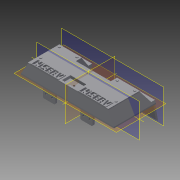
# Autodesk Inventor part: ChassisHintenUnten
Saved by Autodesk Inventor 2015 (Build 190159000, 159)
## iProperties
Created: 2018-11-28
Part Number: ChassisHintenUnten
Material: Generisch
Document SubType Name: Modeling
Designer: Boris
Density: 1 g/cm^3
Appearance: Vorgabe
Author: Boris
Autodesk Inventor part; units mm, degrees
sketch "Skizze1" plane through (0, 0, 0) normal (0, 0, 1) x (1, 0, 0)
  line L0 (-76, 34.5) -> (76, 34.5)
  line L1 (76, 34.5) -> (76, -34.5)
  line L2 (76, -34.5) -> (-76, -34.5)
  line L3 (-76, -34.5) -> (-76, 34.5)
  line L4 (0, -48.3) -> (0, 48.3) projected
  line L5 (-106.4, 0) -> (106.4, 0) projected
  point P0 (0, 0)
  dimension "d0" = 69
  dimension "d1" = 152
  constraints: 8 end point, 2 parallel, 1 horizontal, 1 perpendicular, 2 other
  measures "d0" distance of L0.end L1.end
  measures "d1" distance of L1.end L2.end
extrude "Extrusion1" add sketch "Skizze1" along normal blind 20
sketch "Skizze2" plane through (0, 0, 20) normal (0, 0, 1) x (1, 0, 0)
  line L0 (-76, 34.5) -> (-76, -34.5) projected
  line L1 (-76, -34.5) -> (76, -34.5) projected
  line L2 (76, -34.5) -> (76, 34.5) projected
  line L3 (-74.5, 34.5) -> (-74.5, -33)
  line L4 (-74.5, -33) -> (74.5, -33)
  line L5 (74.5, -33) -> (74.5, 34.5)
  line L6 (-76, 34.5) -> (-74.5, 34.5)
  line L7 (76, 34.5) -> (-76, 34.5) projected
  line L8 (74.5, 34.5) -> (76, 34.5)
  point P0 (0, 0)
  dimension "d4" = 1.5
  constraints: 10 end point, 1 collinear, 1 horizontal, 2 other
  measures "d4" distance between parallel lines of L0 L3
extrude "Extrusion2" cut sketch "Skizze2" against normal blind 20 contours L6 L3 L4 L5 L7 L2 L1 L0
sketch "Skizze4" plane through (0, 0, 20) normal (0, 0, 1) x (1, 0, 0)
  line L0 (-74.5, 34.5) -> (-74.5, -33) projected
  line L1 (-74.5, -33) -> (74.5, -33) projected
  line L2 (74.5, -33) -> (74.5, 34.5) projected
  line L3 (74.5, 34.5) -> (-74.5, 34.5) projected
  line L4 (-74.5, 34.5) -> (74.5, 34.5)
  line L5 (74.5, 34.5) -> (74.5, 28.5)
  line L6 (74.5, 28.5) -> (-74.5, 28.5)
  line L7 (-74.5, 28.5) -> (-74.5, 34.5)
  point P0 (0, 0)
  dimension "d10" = 6
  constraints: 8 end point, 2 parallel, 1 horizontal, 1 perpendicular, 1 point on line
  measures "d10" distance of L4.end L5.end
extrude "Extrusion4" cut sketch "Skizze4" against normal blind 15 contours L3 L2 L6 L0
chamfer "Fase1" distance 10 distance2 15 1 edges at (0, 28.5, 20) measured on face at (0, 28, 20)
chamfer "Fase2" distance 1 distance2 18 1 edges at (0, -33, 20) measured on face at (0, -32.5, 20)
sketch "Skizze5" plane through (-76, -34.5, 0) normal (-1, 0, 0) x (0, 0, 1)
  line L0 (0, 88.3544) -> (0, -14.7257) projected
  line L1 (0, 69) -> (-26.5167, 73.8189)
  line L2 (0, 69) -> (26.951, 69) construction
  line L3 (-26.5167, 73.8189) -> (-23.2032, 70.2167)
  line L4 (-26.5167, 73.8189) -> (-22.013, 73.8189) construction
  line L5 (0, 69) -> (0, 66)
  line L6 (0, 0) -> (0, 69) projected
  line L7 (0, 66) -> (-23.2032, 70.2167)
  point P0 (0, 34.5)
  dimension "d19" = 169.7
  dimension "d21" = 26.951
  dimension "d22" = 47.39
  dimension "d23" = 3
  constraints: 12 end point, 2 horizontal, 1 equal length, 1 parallel, 1 point on line
  measures "d19" angle of L2 L1
  measures "d21" distance of L1.start L1.end
  measures "d22" angle of L3 L4
  measures "d23" distance of L1.start L5.end
extrude "Extrusion5" add sketch "Skizze5" against normal up to surface (152 mm away)
fillet "Rundung1" radius 2 1 edges at (0, 31.5, 0)
sketch "Skizze6" plane through (0, 0, 20) normal (0, 0, 1) x (1, 0, 0)
  line L0 (-28, 46.7837) -> (28, 46.7837)
  line L1 (28, 46.7837) -> (28, 8.5)
  line L2 (28, 8.5) -> (-28, 8.5)
  line L3 (-28, 8.5) -> (-28, 46.7837)
  line L4 (0, 63.0404) -> (0, -50.7567) projected
  line L5 (-74.5, 18.5) -> (74.5, 18.5) projected
  point P0 (0, 0)
  dimension "d27" = 56
  dimension "d28" = 10
  constraints: 8 end point, 2 parallel, 1 horizontal, 1 perpendicular, 1 other
  measures "d27" distance of L1.end L2.end
  measures "d28" distance between parallel lines of L2 L5
extrude "Extrusion6" cut sketch "Skizze6" against normal blind 10
chamfer "Fase3" distance 10 distance2 18 1 edges at (74.5, -6.75, 20) measured on face at (74, -6.75, 20)
chamfer "Fase4" distance 10 distance2 18 1 edges at (-74.5, -6.75, 20) measured on face at (-74, -6.75, 20)
sketch "Skizze7" plane through (0, 0, 0) normal (0, 0, -1) x (-1, 0, 0)
  line L0 (-74.5, 29.8307) -> (74.5, 29.8307) projected
  line L1 (69, 22.8307) -> (-69, 22.8307)
  line L2 (-69, 22.8307) -> (-69, -27.5)
  line L3 (-69, -27.5) -> (69, -27.5)
  line L4 (69, -27.5) -> (69, 22.8307)
  line L5 (-74.5, 29.8307) -> (-74.5, -33) projected
  line L6 (-74.5, -33) -> (74.5, -33) projected
  line L7 (74.5, -33) -> (74.5, 29.8307) projected
  point P0 (0, 0)
  dimension "d37" = 7
  constraints: 8 end point
  measures "d37" distance between parallel lines of L0 L1
extrude "Extrusion7" cut sketch "Skizze7" against normal blind 10 contours L4 L3 L2 L1
sketch "Skizze8" plane through (0, 0, 10) normal (0, 0, -1) x (-1, 0, 0)
  line L0 (60.5, -27.5) -> (-60.5, -27.5)
  line L1 (-60.5, -32) -> (-60.5, 14.5)
  line L2 (-60.5, 14.5) -> (-32, 14.5)
  line L3 (-32, 14.5) -> (-32, 4.5)
  line L4 (-32, 4.5) -> (32, 4.5)
  line L5 (32, 4.5) -> (32, 14.5)
  line L6 (32, 14.5) -> (60.5, 14.5)
  line L7 (60.5, 14.5) -> (60.5, -32)
  point P0 (0, 0)
  point P1 (-28, 18.5)
  point P2 (28, 8.5)
  point P3 (-64.5, 28.5)
  point P4 (64.5, 28.5)
  constraints: 16 end point, 2 point on line
extrude "Extrusion8" cut sketch "Skizze8" against normal blind 4
sketch "Skizze9" plane through (0, 0, 10) normal (0, 0, 1) x (1, 0, 0)
  line L0 (-28, 8.5) -> (-28, 25.1667) projected
  line L1 (-28, 18.5) -> (28, 18.5)
  line L2 (28, 18.5) -> (28, 68.5)
  line L3 (28, 68.5) -> (-28, 68.5)
  line L4 (-28, 68.5) -> (-28, 18.5)
  line L5 (28, 8.5) -> (-28, 8.5) projected
  point P0 (0, 0)
  point P1 (-28, 28.5)
  dimension "d43" = 56
  dimension "d44" = 50
  dimension "d47" = 10
  constraints: 8 end point, 2 parallel, 1 horizontal, 1 perpendicular, 1 point on line
  measures "d43" distance of L3.end L2.end
  measures "d44" distance of L2.end L1.end
  measures "d47" distance between parallel lines of L5 L1
extrude "Extrusion9" cut sketch "Skizze9" against normal blind 60
sketch "Skizze10" plane through (0, 0, 0) normal (0, 0, -1) x (-1, 0, 0)
  line L0 (0, -48.3) -> (0, 48.3) projected
  line L1 (-40, -29.55) -> (-20, -29.55)
  line L2 (-20, -29.55) -> (-20, -32.45)
  line L3 (-20, -32.45) -> (-40, -32.45)
  line L4 (-40, -32.45) -> (-40, -29.55)
  point P0 (0, 0)
  dimension "d48" = 20
  dimension "d49" = 2.9
  dimension "d50" = 20
  constraints: 8 end point, 2 parallel, 1 horizontal, 1 perpendicular
  measures "d48" distance of L2.end L3.end
  measures "d49" distance of L1.end L2.end
  measures "d50" distance between parallel lines of L0 L2
extrude "Extrusion10" add sketch "Skizze10" along normal blind 15
fillet "Rundung2" radius 2 2 edges at (40, -31, -15) (20, -31, -15)
sketch "Skizze11" plane through (20, -29.55, 0) normal (0, 1, 0) x (1, 0, 0)
  circle A0 centre (15, 7.5) radius 1.5
  line L0 (20, 0) -> (0, 0) projected
  line L1 (20, 0) -> (20, 13) projected
  line L2 (2, 15) -> (18, 15) projected
  line L3 (10, 15) -> (10, 0)
  circle A1 centre (5, 7.5) radius 1.5
  point P0 (-20, 0)
  dimension "d55" = 3
  dimension "d56" = 7.5
  dimension "d57" = 5
  constraints: 2 centre point, 2 end point, 2 midpoint, 1 symmetric about line, 1 other
  measures "d55" diameter of A0
  measures "d56" distance from line of L0 A0.centre
  measures "d57" distance from line of A0.centre L1
extrude "Extrusion11" cut sketch "Skizze11" against normal blind 15
thread "Gewinde1" size "M3x0.5" class "6H" standard "ANSI Metric M Profile" full length
thread "Gewinde2" size "M3x0.5" class "6H" standard "ANSI Metric M Profile" full length
mirror "Spiegeln1" about plane through (0, 0, 0) normal (1, 0, 0) of "Extrusion10", "Rundung2", "Extrusion11"
sketch "Skizze12" plane through (0, 0, 20) normal (0, 0, 1) x (1, 0, 0)
  line L0 (-64.5, -32) -> (-64.5, 18.5) projected
  line L1 (64.5, -32) -> (-64.5, -32) projected
  line L2 (64.5, 18.5) -> (64.5, -32) projected
  line L3 (28, 18.5) -> (28, 8.5) projected
  line L4 (28, 8.5) -> (-28, 8.5) projected
  line L5 (-28, 8.5) -> (-28, 18.5) projected
  line L6 (28, 18.5) -> (64.5, 18.5) projected
  line L7 (-64.5, 18.5) -> (-28, 18.5) projected
  point P0 (0, 0)
extrude "Extrusion12" add sketch "Skizze12" along normal blind 1.5
sketch "Skizze13" plane through (0, 0, 21.5) normal (0, 0, 1) x (1, 0, 0)
  line L0 (0, 53.7827) -> (0, -47.4638) projected
  line L1 (-106.4, 0) -> (106.4, 0) projected
  line L2 (-64.5, 18.5) -> (-64.5, -32) projected
  line L3 (-64.5, -32) -> (64.5, -32) projected
  line L4 (64.5, -32) -> (64.5, 18.5) projected
  line L5 (28, 18.5) -> (28, 8.5) projected
  line L6 (28, 8.5) -> (-28, 8.5) projected
  line L7 (-28, 8.5) -> (-28, 18.5) projected
  line L8 (-60.5, 14.5) -> (-60.5, -27.5) projected
  line L9 (-60.5, -20) -> (-15.5, -20)
  line L10 (-15.5, -20) -> (-15.5, -32)
  line L11 (-15.5, -32) -> (-60.5, -32)
  line L12 (-60.5, -32) -> (-60.5, -20)
  line L13 (64.5, 18.5) -> (28, 18.5) projected
  line L14 (-28, 18.5) -> (-64.5, 18.5) projected
  point P0 (0, 0)
  dimension "d66" = 45
  dimension "d67" = 12
  dimension "d68" = 0
  constraints: 8 end point, 2 parallel, 1 horizontal, 1 perpendicular, 1 point on line
  measures "d66" distance of L10.end L11.end
  measures "d67" distance of L9.end L10.end
  measures "d68" distance between parallel lines of L3 L11
extrude "Extrusion13" add sketch "Skizze13" along normal blind 1 contours L3 L12 L8 L9 L10
sketch "Skizze14" plane through (0, 0, 22.5) normal (0, 0, 1) x (1, 0, 0)
  line L0 (-15.5, -20) -> (-60.5, -20) projected
  line L1 (-60.5, -20) -> (-60.5, -32) projected
  line L2 (-60.5, -32) -> (-15.5, -32) projected
  line L3 (-15.5, -32) -> (-15.5, -20) projected
  line L4 (-59, -21) -> (-56, -21)
  line L5 (-56, -31) -> (-59, -31)
  line L6 (-59, -31) -> (-59, -21)
  line L7 (-56, -23.9914) -> (-54, -23.9914)
  line L8 (-54, -28.5036) -> (-56, -28.5036)
  line L9 (-54, -21) -> (-51, -21)
  line L10 (-51, -21) -> (-51, -31)
  line L11 (-51, -31) -> (-54, -31)
  line L12 (-56, -21) -> (-56, -23.9914)
  line L13 (-56, -28.5036) -> (-56, -31)
  line L14 (-54, -31) -> (-54, -28.5036)
  line L15 (-54, -23.9914) -> (-54, -21)
  line L16 (-50, -23.25) -> (-47.5, -23.25)
  line L17 (-47.5, -23.25) -> (-47.5, -31)
  line L18 (-47.5, -31) -> (-50, -31)
  line L19 (-50, -31) -> (-50, -23.25)
  circle A0 centre (-48.75, -21.75) radius 0.75
  line L20 (-46.5, -25.4992) -> (-46.5, -23.055)
  line L21 (64.5, -32) -> (-64.5, -32) projected
  arc A1 (-44.8577, -20.9215) -> (-46.5, -23.0565) centre (-44.2912, -23.0565) ccw
  arc A2 (-46.5, -25.4992) -> (-44.9997, -26.9993) centre (-44.9999, -25.4992) ccw
  arc A3 (-43.0091, -27.9051) -> (-44.1074, -26.9992) centre (-44.1072, -28.1176) ccw
  arc A4 (-44.1063, -28.9992) -> (-43.0093, -28.0963) centre (-44.1064, -27.8812) ccw
  line L22 (-44.0918, -28.9991) -> (-46.5, -28.9991)
  line L23 (-46.5, -28.9991) -> (-46.5, -31.0955)
  line L24 (-46.5, -31.0955) -> (-41.2733, -31.0955)
  arc A5 (-43.0093, -28.0963) -> (-43.0091, -27.9051) centre (-43.5, -28.0001) ccw
  line L25 (-38.8577, -21) -> (-32.8577, -21)
  line L26 (-32.8577, -31) -> (-38.8577, -31)
  line L27 (-38.8577, -31) -> (-38.8577, -21)
  line L28 (-32.8577, -23) -> (-35.8577, -23)
  line L29 (-35.0809, -21) -> (-32.8577, -21)
  line L30 (-32.8577, -21) -> (-32.8577, -23)
  line L31 (-32.8577, -25) -> (-35.8577, -25)
  line L32 (-35.8577, -27.2739) -> (-32.8577, -27.2739)
  line L33 (-32.8577, -27.2739) -> (-32.8577, -25)
  line L34 (-32.8577, -31) -> (-35.0862, -31)
  line L35 (-35.8577, -28.799) -> (-32.8577, -28.799)
  line L36 (-32.8577, -28.799) -> (-32.8577, -31)
  line L37 (-44.8577, -20.9215) -> (-39.8577, -20.9215)
  line L38 (-39.8577, -20.9215) -> (-39.8577, -22.9215)
  line L39 (-39.8577, -20.9215) -> (-37.8577, -20.9215) construction
  line L40 (-39.8577, -22.9215) -> (-42.2156, -22.9215)
  line L41 (-39.8577, -22.9215) -> (-33.2733, -22.9215) construction
  line L42 (-42.2207, -25.0955) -> (-41.2733, -25.0955)
  line L43 (-39.7733, -26.5955) -> (-39.7733, -29.5955)
  arc A6 (-41.2733, -31.0955) -> (-39.7733, -29.5955) centre (-41.2733, -29.5955) ccw
  arc A7 (-39.7733, -26.5955) -> (-41.2733, -25.0955) centre (-41.2733, -26.5955) ccw
  arc A8 (-43.5829, -24.2236) -> (-42.2207, -25.0955) centre (-42.2207, -23.5955) ccw
  arc A9 (-42.2156, -22.9215) -> (-43.5855, -23.8105) centre (-42.2156, -24.4215) ccw
  arc A10 (-43.5855, -23.8105) -> (-43.5829, -24.2236) centre (-43.1289, -24.0142) ccw
  line L44 (-32.8577, -21) -> (-32.8577, -23)
  line L45 (-32.8577, -25) -> (-32.8577, -27.2739)
  line L46 (-32.8577, -28.799) -> (-32.8577, -31)
  line L47 (-35.8577, -23) -> (-35.8577, -25)
  line L48 (-35.8577, -27.2739) -> (-35.8577, -28.799)
  line L49 (-31.8577, -21) -> (-26.8577, -21)
  line L50 (-24.8577, -23) -> (-24.8577, -25)
  line L51 (-31.8577, -31) -> (-31.8577, -21)
  line L52 (-27.3577, -31) -> (-27.3577, -27.198)
  line L53 (-27.3577, -27.198) -> (-29.3577, -27.198)
  line L54 (-29.3577, -27.198) -> (-29.3577, -31)
  arc A11 (-24.8577, -23) -> (-26.8577, -21) centre (-26.8577, -23) ccw
  line L55 (-46.5, -25.4992) -> (-46.5, -23.0565)
  line L56 (-46.5, -23.055) -> (-46.5028, -25.0955)
  line L57 (-46.5057, -27.198) -> (-46.5058, -27.2739)
  line L58 (-28.6122, -25.0924) -> (-27.6122, -25.0924)
  line L59 (-26.6122, -24.0924) -> (-26.6122, -23.9819)
  line L60 (-27.6122, -22.9819) -> (-28.6122, -22.9819)
  line L61 (-28.6122, -22.9819) -> (-28.6122, -25.0924)
  arc A12 (-26.6122, -23.9819) -> (-27.6122, -22.9819) centre (-27.6122, -23.9819) ccw
  arc A13 (-27.6122, -25.0924) -> (-26.6122, -24.0924) centre (-27.6122, -24.0924) ccw
  arc A14 (-25.8131, -25.999) -> (-24.8577, -25) centre (-25.8577, -25) ccw
  line L62 (-24.8577, -31) -> (-24.8577, -26.998)
  arc A15 (-24.8577, -26.998) -> (-25.8131, -25.999) centre (-25.8577, -26.998) ccw
  line L63 (-24.8577, -31) -> (-27.3577, -31)
  line L64 (-29.3577, -31) -> (-31.8577, -31)
  line L65 (-21.2706, -31) -> (-18.7095, -31)
  line L66 (-18.7095, -31) -> (-16.2095, -21)
  line L67 (-16.2095, -21) -> (-18.7095, -21)
  line L68 (-18.7095, -21) -> (-19.9901, -26.1223)
  line L69 (-19.9901, -26.1223) -> (-21.2706, -21)
  line L70 (-21.2706, -21) -> (-23.7706, -21)
  line L71 (-23.7706, -21) -> (-21.2706, -31)
  line L72 (-44.9997, -26.9993) -> (-44.1074, -26.9992)
  point P0 (0, 0)
  point P1 (-46.5, -26.9995)
  point P2 (-46.5, -28.9995)
  dimension "d71" = 3
  dimension "d72" = 1.5
  dimension "d73" = 1
  dimension "d74" = 1
  dimension "d77" = 1
  dimension "d78" = 1
  dimension "d79" = 1.5
  dimension "d80" = 1.5
  dimension "d81" = 1
  dimension "d82" = 2.5
  dimension "d83" = 0.5
  dimension "d95" = 0.5
  dimension "d96" = 6
  dimension "d99" = 1
  dimension "d100" = 1
  dimension "d102" = 3
  dimension "d103" = 2
  dimension "d104" = 2
  dimension "d105" = 3
  dimension "d113" = 1.5
  dimension "d114" = 3
  dimension "d115" = 0.5
  dimension "d116" = 5
  dimension "d117" = 2
  dimension "d118" = 3
  dimension "d119" = 5.2267
  dimension "d120" = 1
  dimension "d121" = 7
  dimension "d122" = 1
  dimension "d123" = 2.5
  dimension "d124" = 2.5
  dimension "d125" = 2
  dimension "d127" = 1
  dimension "d128" = 2.8712
  dimension "d129" = 1
  dimension "d130" = 1
  dimension "d131" = 3
  dimension "d132" = 3
  dimension "d133" = 1
  dimension "d134" = 1
  dimension "d135" = 1
  dimension "d136" = 3
  dimension "d137" = 2.5
  dimension "d138" = 2.5
  dimension "d140" = 0
  dimension "d141" = 0
  dimension "d142" = 1
  dimension "d143" = 1
  dimension "d144" = 1
  constraints: 136 end point, 32 point on circle, 28 parallel, 23 tangent, 16 centre point, 16 horizontal, 14 perpendicular, 11 point on line, 3 equal radius, 1 vertical
  measures "d71" distance of L4.start L4.end
  measures "d72" distance between parallel lines of L1 L6
  measures "d73" distance between parallel lines of L2 L5
  measures "d74" distance between parallel lines of L4 L0
  measures "d77" distance between parallel lines of L2 L18
  measures "d78" distance between parallel lines of L10 L19
  measures "d79" distance from line of L16 A0.centre
  measures "d80" diameter of A0
  measures "d81" distance edge to line of A0 L0
  measures "d82" distance of L17.end L18.end
  measures "d83" distance edge to line of A0 L19
  measures "d95" radius of A5
  measures "d96" distance of L25.start L25.end
  measures "d99" distance between parallel lines of L17 L23
  measures "d100" distance between parallel lines of L17 L20
  measures "d102" distance of L9.start L9.end
  measures "d103" distance of L7.start L7.end
  measures "d104" distance of L8.start L8.end
  measures "d105" distance from line of L23 A5.centre
  measures "d113" radius of A6
  measures "d114" diameter of A9
  measures "d115" radius of A10
  measures "d116" distance of L37.start L37.end
  measures "d117" distance of L37.end L38.end
  measures "d118" distance of L43.start L43.end
  measures "d119" distance of L23.end L24.end
  measures "d120" distance between parallel lines of L38 L27
  measures "d121" distance of L62.start L51.start
  measures "d122" distance between parallel lines of L51 L30
  measures "d123" distance between parallel lines of L51 L54
  measures "d124" distance between parallel lines of L50 L52
  measures "d125" radius of A11
  measures "d127" distance between parallel lines of L17 L55
  measures "d128" distance edge to line of A10 L55
  measures "d129" distance between parallel lines of L51 L33
  measures "d130" distance between parallel lines of L51 L36
  measures "d131" distance between parallel lines of L27 L47
  measures "d132" distance between parallel lines of L27 L48
  measures "d133" radius of A12
  measures "d134" radius of A14
  measures "d135" radius of A15
  measures "d136" distance of L10.end L11.end
  measures "d137" distance of L69.end L70.end
  measures "d138" distance of L66.end L67.end
  measures "d140" horizontal distance of L65.start L69.end
  measures "d141" horizontal distance of L65.end L67.end
  measures "d142" distance between parallel lines of L2 L64
  measures "d143" distance between parallel lines of L0 L49
  measures "d144" distance between parallel lines of L21 L63
extrude "Extrusion14" cut sketch "Skizze14" against normal blind 3 contours L4 L12 L7 L15 L9 L10 L11 L14 L8 L13 L5 L6 | L16 L17 L18 L19 | A0 | L20 A1 L37 L38 L40 A9 A10 A8 L42 A7 L43 A6 L24 L23 L22 A4 A5 A3 L72 A2 | L25 L30 L28 L47 L31 L33 L32 L48 L35 L36 L26 L27 | L49 A11 L50 A14 A15 L62 L63 L52 L53 L54 L64 L51 | L71 L70 L69 L68 L67 L66 L65
pattern_linear "Rechteckige Anordnung1" count 2 spacing 76 along (1, 0, 0) of "Extrusion13", "Extrusion14"
sketch "Skizze17" plane through (-76, -34.5, 0) normal (-1, 0, 0) x (0, 0, 1)
  arc A0 (0, 64.3307) -> (-1.6424, 66.2985) centre (-2, 64.3307) ccw projected
  line L0 (-26.5167, 73.8189) -> (-23.2032, 70.2167)
  line L1 (-23.2032, 70.2167) -> (-1.6424, 66.2985)
  arc A1 (0, 64.3307) -> (-1.6424, 66.2985) centre (-2, 64.3307) ccw projected
  line L2 (0, 64.3307) -> (0, 69)
  line L3 (0, 69) -> (0, 66) projected
  line L4 (0, 69) -> (-26.5167, 73.8189)
  line L5 (0, 69) -> (-26.5167, 73.8189) projected
  point P0 (0, 34.5)
  constraints: 8 end point, 2 collinear, 1 tangent
extrude "Extrusion17" cut sketch "Skizze17" against normal blind 3
mirror "Spiegeln3" about plane through (0, 0, 0) normal (1, 0, 0) of "Extrusion17"
sketch "Skizze18" plane through (0, 0, 21.5) normal (0, 0, 1) x (1, 0, 0)
  line L0 (0, 53.7827) -> (0, -47.4638) projected
  line L1 (-104.3, 0) -> (104.3, 0) projected
  line L2 (-12.75, -15.5) -> (12.75, -15.5)
  line L3 (12.75, -15.5) -> (12.75, -29)
  line L4 (12.75, -29) -> (-12.75, -29)
  line L5 (-12.75, -29) -> (-12.75, -15.5)
  line L6 (-15.5, -32) -> (15.5, -32) projected
  point P0 (0, 0)
  dimension "d157" = 25.5
  dimension "d158" = 13.5
  dimension "d159" = 3
  constraints: 8 end point, 2 parallel, 1 horizontal, 1 perpendicular, 1 other
  measures "d157" distance of L3.end L4.end
  measures "d158" distance of L2.end L3.end
  measures "d159" distance between parallel lines of L6 L4
extrude "Extrusion18" cut sketch "Skizze18" against normal blind 5 draft 8
sketch "Skizze19" plane through (0, 0, 16.5) normal (0, 0, 1) x (1, 0, 0)
  line L0 (0, 53.7827) -> (0, -47.4638) projected
  circle A0 centre (0, -22.25) radius 1.5
  line L1 (12.75, -29) -> (-12.75, -29) projected
  point P0 (0, 0)
  dimension "d162" = 3
  dimension "d163" = 6.75
  constraints: 1 centre point, 1 point on line
  measures "d162" diameter of A0
  measures "d163" distance from line of L1 A0.centre
extrude "Extrusion19" cut sketch "Skizze19" against normal blind 3
sketch "Skizze20" plane through (0, 0, 14) normal (0, 0, -1) x (-1, 0, 0)
  circle A0 centre (0, -22.25) radius 1.5 projected
  line L0 (0, -19.25) -> (2.5981, -20.75)
  line L1 (2.5981, -20.75) -> (2.5981, -23.75)
  line L2 (2.5981, -23.75) -> (0, -25.25)
  line L3 (0, -25.25) -> (-2.5981, -23.75)
  line L4 (-2.5981, -23.75) -> (-2.5981, -20.75)
  line L5 (-2.5981, -20.75) -> (0, -19.25)
  point P0 (0, 0)
  constraints: 12 end point, 1 coincident, 13 other
extrude "Extrusion20" cut sketch "Skizze20" against normal blind 1
ref_plane "Arbeitsebene1" through (-73, 39.3189, -26.5167) normal (0, 1, 0) x (-1, 0, 0)
sketch "Skizze21" plane through (-73, 39.3189, -26.5167) normal (0, 1, 0) x (-1, 0, 0)
  circle A0 centre (-9, 21.5167) radius 1.45
  line L0 (0, 0) -> (0, 26.5167) projected
  line L1 (0, 26.5167) -> (-45, 26.5167) projected
  line L2 (-73, -9.8033) -> (-73, 58.82) projected
  circle A1 centre (-137, 21.5167) radius 1.45
  point P0 (-73, 26.5167)
  dimension "d169" = 2.9
  dimension "d170" = 9
  dimension "d171" = 5
  constraints: 2 centre point, 1 symmetric about line, 1 other
  measures "d169" diameter of A0
  measures "d170" distance from line of L0 A0.centre
  measures "d171" distance from line of L1 A0.centre
extrude "Extrusion21" cut sketch "Skizze21" against normal blind 10
thread "Gewinde3" size "M3x0.5" class "6H" standard "ANSI Metric M Profile" full length
thread "Gewinde4" size "M3x0.5" class "6H" standard "ANSI Metric M Profile" full length
sketch "Skizze22" plane through (0, 0, 21.5) normal (0, 0, 1) x (1, 0, 0)
  line L0 (0, 53.7827) -> (0, -47.4638) projected
  line L1 (-28, 18.5) -> (-64.5, 18.5) projected
  line L2 (-64.5, 18.5) -> (-64.5, -32) projected
  line L3 (-60.5, 16.5) -> (-58.7679, 15.5)
  line L4 (-58.7679, 15.5) -> (-58.7679, 13.5)
  line L5 (-58.7679, 13.5) -> (-60.5, 12.5)
  line L6 (-60.5, 12.5) -> (-62.2321, 13.5)
  line L7 (-62.2321, 13.5) -> (-62.2321, 15.5)
  line L8 (-62.2321, 15.5) -> (-60.5, 16.5)
  line L9 (-60.5, -13.5) -> (-58.7679, -14.5)
  line L10 (-58.7679, -14.5) -> (-58.7679, -16.5)
  line L11 (-58.7679, -16.5) -> (-60.5, -17.5)
  line L12 (-60.5, -17.5) -> (-62.2321, -16.5)
  line L13 (-62.2321, -16.5) -> (-62.2321, -14.5)
  line L14 (-62.2321, -14.5) -> (-60.5, -13.5)
  line L15 (-32.5, 16.5) -> (-30.7679, 15.5)
  line L16 (-30.7679, 15.5) -> (-30.7679, 13.5)
  line L17 (-30.7679, 13.5) -> (-32.5, 12.5)
  line L18 (-32.5, 12.5) -> (-34.2321, 13.5)
  line L19 (-34.2321, 13.5) -> (-34.2321, 15.5)
  line L20 (-34.2321, 15.5) -> (-32.5, 16.5)
  line L21 (60.5, 16.5) -> (58.7679, 15.5)
  line L22 (58.7679, 15.5) -> (58.7679, 13.5)
  line L23 (58.7679, 13.5) -> (60.5, 12.5)
  line L24 (60.5, 12.5) -> (62.2321, 13.5)
  line L25 (62.2321, 13.5) -> (62.2321, 15.5)
  line L26 (62.2321, 15.5) -> (60.5, 16.5)
  line L27 (62.2321, -14.5) -> (60.5, -13.5)
  line L28 (62.2321, -16.5) -> (62.2321, -14.5)
  line L29 (60.5, -17.5) -> (62.2321, -16.5)
  line L30 (58.7679, -16.5) -> (60.5, -17.5)
  line L31 (58.7679, -14.5) -> (58.7679, -16.5)
  line L32 (60.5, -13.5) -> (58.7679, -14.5)
  line L33 (32.5, 16.5) -> (30.7679, 15.5)
  line L34 (34.2321, 15.5) -> (32.5, 16.5)
  line L35 (34.2321, 13.5) -> (34.2321, 15.5)
  line L36 (32.5, 12.5) -> (34.2321, 13.5)
  line L37 (30.7679, 13.5) -> (32.5, 12.5)
  line L38 (30.7679, 15.5) -> (30.7679, 13.5)
  point P0 (0, 0)
  point P1 (-60.5, 14.5)
  dimension "d183" = 30
  dimension "d190" = 28
  constraints: 72 end point, 18 symmetric about line, 1 horizontal, 1 vertical, 37 other
  measures "d183" distance of L7.end L14.start
  measures "d190" distance of L3.start L15.start
extrude "Extrusion22" add sketch "Skizze22" along normal blind 1
